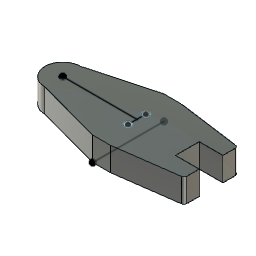
wing_interface_v2 v6 (Autodesk Fusion 360 design; units mm, degrees)
Autodesk Fusion 360 part; units mm, degrees
sketch "Sketch1" plane through (0, 0, 0) normal (0, 0, 1) x (1, 0, 0)
  line L0 (25, -3) -> (25, 3)
  circle A0 centre (0, 0) radius 0.5
  line L1 (25, 0) -> (21, 0)
  line L2 (21, 0) -> (21, -2)
  line L3 (21, -2) -> (25, -2)
  line L4 (25, -2) -> (25, 0)
  line L5 (25, 0) -> (11, 0)
  line L6 (25, 4.5) -> (25, 0)
  line L7 (11, 0) -> (25, 0)
  line L8 (25, 0) -> (25, -4.5)
  line L9 (25, 0) -> (21, 0)
  line L10 (21, 0) -> (21, 2)
  line L11 (21, 2) -> (25, 2)
  line L12 (25, 2) -> (25, 0)
  line L13 (25, -2) -> (21, -2)
  line L14 (25, -4.5) -> (25, -2)
  line L15 (25, 2) -> (21, 2)
  line L16 (25, 4.5) -> (25, 2)
  line L17 (0, 3) -> (11, 6)
  line L18 (0, -3) -> (11, -6)
  line L19 (11, -6) -> (14, -6)
  line L20 (14, -6) -> (25, -4.5)
  line L21 (11, 6) -> (14, 6)
  line L22 (14, 6) -> (25, 4.5)
  arc A1 (0, 3) -> (0, -3) centre (0, 0) ccw
  dimension "d1" = 6
  dimension "d3" = 1
  constraint coincident A0.centre A1.centre
  constraint vertical L0
  constraint horizontal L1
  constraint vertical L2
  constraint horizontal L3
  constraint vertical L4
  constraint midpoint L0 L1.start
  constraint horizontal L5
  constraint vertical L6
  constraint horizontal L7
  constraint vertical L8
  constraint horizontal L9
  constraint vertical L10
  constraint horizontal L11
  constraint vertical L12
  constraint horizontal L13
  constraint vertical L14
  constraint horizontal L15
  constraint vertical L16
  measures "d1" diameter of A1
  measures "d3" diameter of A0
extrude "Extrude1" add sketch "Sketch1" along normal blind 4 contours L0 L2 L3 L6 L8 L10 L11 L13 L14 L15 L16 L17 L18 L19 L20 L21 L22 A1
fillet "Fillet1" radius 0.5 1 edges at (25, -4.5, 2)
fillet "Fillet2" radius 0.5 1 edges at (25, 4.5, 2)
fillet "Fillet3" radius 0.5 1 edges at (14, 6, 2)
fillet "Fillet4" radius 0.5 1 edges at (11, 6, 2)
fillet "Fillet5" radius 0.5 1 edges at (14, -6, 2)
fillet "Fillet6" radius 0.5 1 edges at (11, -6, 2)
sketch "Sketch2" plane through (0, 0, 0) normal (0, 0, 1) x (1, 0, 0)
sketch "Sketch3" plane through (0, 0, 0) normal (0, 1, 0) x (1, 0, 0)
sketch "Sketch6" plane through (0, 0, 0) normal (0, 0, -1) x (1, 0, 0)
  circle A0 centre (0, 0) radius 0.5
  arc A1 (11.067, 6) -> (10.9354, 5.9824) centre (11.067, 5.5) ccw
  line L0 (10.9354, 5.9824) -> (0, 3)
  arc A2 (0, 3) -> (0, -3) centre (0, 0) ccw
  line L1 (0, -3) -> (10.9354, -5.9824)
  arc A3 (10.9354, -5.9824) -> (11.067, -6) centre (11.067, -5.5) ccw
  line L2 (11.067, -6) -> (13.9661, -6)
  arc A4 (13.9661, -6) -> (14.0336, -5.9954) centre (13.9661, -5.5) ccw
  line L3 (14.0336, -5.9954) -> (24.5676, -4.559)
  arc A5 (24.5676, -4.559) -> (25, -4.0636) centre (24.5, -4.0636) ccw
  line L4 (25, -4.0636) -> (25, -2)
  line L5 (25, -2) -> (21, -2)
  line L6 (21, -2) -> (21, 2)
  line L7 (21, 2) -> (25, 2)
  line L8 (25, 2) -> (25, 4.0636)
  arc A6 (25, 4.0636) -> (24.5676, 4.559) centre (24.5, 4.0636) ccw
  line L9 (24.5676, 4.559) -> (14.0336, 5.9954)
  arc A7 (14.0336, 5.9954) -> (13.9661, 6) centre (13.9661, 5.5) ccw
  line L10 (13.9661, 6) -> (11.067, 6)
  line L11 (11.067, 6) -> (11.067, -6)
  dimension "d22" = 21
  constraint coincident A1.start L10.end
  constraint coincident A3.end L2.start
  measures "d22" distance of A0.centre L6
sketch "Sketch7" plane through (0, 0, 4) normal (0, 0, 1) x (-1, 0, 0)
  arc A0 (-10.9354, 5.9824) -> (-11.067, 6) centre (-11.067, 5.5) ccw
  line L0 (-11.067, 6) -> (-13.9661, 6)
  arc A1 (-13.9661, 6) -> (-14.0336, 5.9954) centre (-13.9661, 5.5) ccw
  line L1 (-14.0336, 5.9954) -> (-24.5676, 4.559)
  arc A2 (-24.5676, 4.559) -> (-25, 4.0636) centre (-24.5, 4.0636) ccw
  line L2 (-25, 4.0636) -> (-25, 2)
  line L3 (-25, 2) -> (-21, 2)
  line L4 (-21, 2) -> (-21, -2)
  line L5 (-21, -2) -> (-25, -2)
  line L6 (-25, -2) -> (-25, -4.0636)
  arc A3 (-25, -4.0636) -> (-24.5676, -4.559) centre (-24.5, -4.0636) ccw
  line L7 (-24.5676, -4.559) -> (-14.0336, -5.9954)
  arc A4 (-14.0336, -5.9954) -> (-13.9661, -6) centre (-13.9661, -5.5) ccw
  line L8 (-13.9661, -6) -> (-11.067, -6)
  arc A5 (-11.067, -6) -> (-10.9354, -5.9824) centre (-11.067, -5.5) ccw
  line L9 (-10.9354, -5.9824) -> (0, -3)
  arc A6 (0, -3) -> (0, 3) centre (0, 0) ccw
  line L10 (0, 3) -> (-10.9354, 5.9824)
  circle A7 centre (0, 0) radius 0.5
  line L11 (0, 0) -> (-12.5, 0)
  line L12 (-12.5, 0) -> (-12.5, -1.5)
  line L13 (-12.5, 0) -> (-12.5, 1.5)
  circle A8 centre (-12.5, -1.5) radius 0.5
  circle A9 centre (-12.5, 1.5) radius 0.5
  dimension "d23" = 12.5
  dimension "d24" = 1
  dimension "d25" = 1
  constraint coincident A6.centre A7.centre
  constraint horizontal L11
  constraint perpendicular L11 L12
  constraint perpendicular L11 L13
  constraint coincident L12.end A8.centre
  constraint coincident L13.end A9.centre
  measures "d23" distance of A6.centre L11.end
  measures "d24" diameter of A8
  measures "d25" diameter of A9
hole "Hole1" at (12.5, 1.5, 4) direction (0, 0, -1) diameter 1 depth 2 tip angle 118
hole "Hole2" at (12.5, -1.5, 4) direction (0, 0, -1) diameter 1 depth 2 tip angle 118
ref_plane "WorkPlane1" through (0, 0, 12) normal (0, 0, 1) x (1, 0, 0)
equation "d25 = mm"
